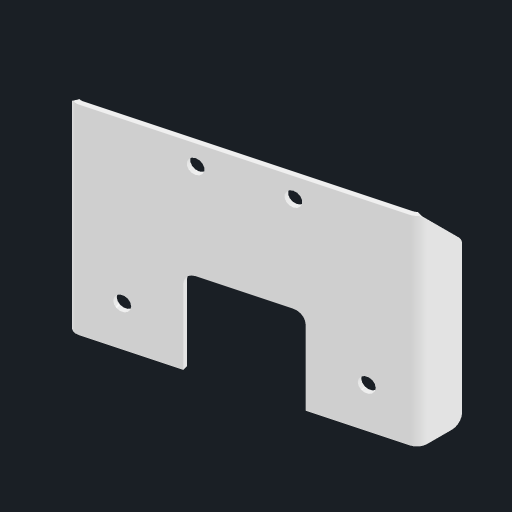
# Autodesk Inventor part: cradle
Saved by Autodesk Inventor 2024.2 (Build 282272000, 272)
## iProperties
Created: 2024-01-06
Part Number: cradle
Material: Generic
Document SubType Name: Sheet Metal
Designer: reima
Density: 1 g/cm^3
Sheet Metal Rule: Default
Appearance: White
Flat Pattern Width: 6.35 cm
Flat Pattern Length: 11.4296 cm
Flat Pattern Area: 72.5782 cm^2
Sheet Metal Width: 2.500 in
Sheet Metal Length: 4.500 in
Sheet Metal Area: 11.250 in^2
Author: reima
Autodesk Inventor part; units mm, degrees
ref_plane "YZ Plane" through (0, 0, 0) normal (1, 0, 0) x (0, 1, 0)
ref_plane "XZ Plane" through (0, 0, 0) normal (0, 1, 0) x (-1, 0, 0)
ref_plane "XY Plane" through (0, 0, 0) normal (0, 0, 1) x (1, 0, 0)
sketch "Sketch1" plane through (0, 0, 0) normal (1, 0, 0) x (0, 1, 0)
  ellipse E0 centre (-29.9633, -76.9903) end of major axis (-32.2747, -76.9903) minor radius 2.3111
  ellipse E1 centre (-29.9633, -102.3866) end of major axis (-32.2747, -102.3866) minor radius 2.3111
  line L0 (-23.6133, -45.2403) -> (-87.1133, -45.2403)
  line L1 (-87.1133, -45.2403) -> (-87.1133, -134.1366)
  line L2 (-87.1133, -134.1366) -> (-23.6133, -134.1366)
  line L3 (-23.6133, -134.1366) -> (-23.6133, -45.2403)
  line L4 (-87.1133, -45.2403) -> (-87.1133, -35.7153)
  line L5 (-87.1133, -45.2403) -> (-77.5883, -45.2403) construction
  line L6 (-23.6133, -45.2403) -> (-35.3834, -33.4702)
  line L7 (-23.6133, -45.2403) -> (-6.9679, -45.2403) construction
  line L8 (-37.6284, -32.5403) -> (-83.9383, -32.5403)
  arc A0 (-83.9383, -32.5403) -> (-87.1133, -35.7153) centre (-83.9383, -35.7153) ccw
  arc A1 (-35.3834, -33.4702) -> (-37.6284, -32.5403) centre (-37.6284, -35.7153) ccw
  line L9 (-87.1133, -89.6885) -> (-23.6133, -89.6885) construction
  line L10 (-87.1133, -134.1366) -> (-87.1133, -143.6616)
  line L11 (-87.1133, -134.1366) -> (-77.5883, -134.1366) construction
  line L12 (-23.6133, -134.1366) -> (-35.3834, -145.9067)
  line L13 (-37.6284, -146.8366) -> (-83.9383, -146.8366)
  arc A2 (-87.1133, -143.6616) -> (-83.9383, -146.8366) centre (-83.9383, -143.6616) ccw
  arc A3 (-37.6284, -146.8366) -> (-35.3834, -145.9067) centre (-37.6284, -143.6616) ccw
  point P0 (0, 0)
  point P1 (-87.1133, -32.5403)
  point P2 (-87.1133, -146.8366)
  dimension "d0" = 6.35
  dimension "d1" = 31.75
  dimension "d2" = 31.75
  dimension "d3" = 63.5
  dimension "d4" = 12.7
  dimension "d5" = 90
  dimension "d6" = 135
  dimension "d7" = 3.175
  measures "d0" distance from line of L3 point (-29.963, -102.387)
  measures "d1" distance from line of point (-29.963, -102.387) L2
  measures "d2" distance from line of point (-29.963, -76.99) L0
  measures "d3" distance between parallel lines of L1 L3
  measures "d4" distance of L0.end point (-87.113, -32.54)
  measures "d5" angle of L5 L4
  measures "d6" angle of L7 L6
  measures "d7" radius of A0
extrude "Plate1" add sketch "Sketch1" along normal blind 1.5875
sketch "Sketch3" plane through (0, 0, 0) normal (-1, 0, 0) x (0, 0, 1)
  ellipse E0 centre (-102.3866, -29.9633) end of major axis (-102.3866, -27.6519) minor radius 2.3111 construction
  ellipse E1 centre (-76.9903, -29.9633) end of major axis (-76.9903, -27.6519) minor radius 2.3111 construction
  arc A0 (-32.5403, -37.6284) -> (-33.4702, -35.3834) centre (-35.7153, -37.6284) ccw construction
  line L0 (-45.2403, -23.6133) -> (-33.4702, -35.3834) construction
  line L1 (-134.1366, -23.6133) -> (-45.2403, -23.6133) construction
  line L2 (-145.9067, -35.3834) -> (-134.1366, -23.6133) construction
  arc A1 (-145.9067, -35.3834) -> (-146.8366, -37.6284) centre (-143.6616, -37.6284) ccw construction
  line L3 (-146.8366, -83.9383) -> (-146.8366, -37.6284) construction
  arc A2 (-146.8366, -83.9383) -> (-143.6616, -87.1133) centre (-143.6616, -83.9383) ccw construction
  line L4 (-35.7153, -87.1133) -> (-143.6616, -87.1133) construction
  arc A3 (-35.7153, -87.1133) -> (-32.5403, -83.9383) centre (-35.7153, -83.9383) ccw construction
  line L5 (-32.5403, -37.6284) -> (-32.5403, -83.9383) construction
  line L6 (-45.2403, -23.6133) -> (-45.2403, -87.1133) construction
  line L7 (-134.1366, -23.6133) -> (-134.1366, -87.1133) construction
  point P0 (0, 0)
  constraints: 4 end point, 2 point on line, 1 perpendicular, 1 vertical
fold "Fold1" angle 75 bend radius 1.5875 thickness 1.5875 k factor 0.44 line from (0, -23.6133, -45.2403) to (0, -87.1133, -45.2403) line at bend centre moving side (0, 0, 1) folds toward (-1, 0, 0)
sketch "Sketch4" plane through (0, 0, 0) normal (-1, 0, 0) x (0, 0, 1)
  line L0 (-46.7365, -87.1133) -> (-46.7365, -23.6133) construction
  line L1 (-134.1366, -23.6133) -> (-46.7365, -23.6133) construction
  line L2 (-145.9067, -35.3834) -> (-134.1366, -23.6133) construction
  arc A0 (-145.9067, -35.3834) -> (-146.8366, -37.6284) centre (-143.6616, -37.6284) ccw construction
  line L3 (-146.8366, -83.9383) -> (-146.8366, -37.6284) construction
  arc A1 (-146.8366, -83.9383) -> (-143.6616, -87.1133) centre (-143.6616, -83.9383) ccw construction
  line L4 (-46.7365, -87.1133) -> (-143.6616, -87.1133) construction
  ellipse E0 centre (-102.3866, -29.9633) end of major axis (-102.3866, -27.6519) minor radius 2.3111 construction
  ellipse E1 centre (-76.9903, -29.9633) end of major axis (-76.9903, -27.6519) minor radius 2.3111 construction
  line L5 (-134.1366, -23.6133) -> (-134.1366, -87.1133)
  point P0 (0, 0)
  constraints: 2 end point, 1 perpendicular, 1 point on line
fold "Fold2" angle 75 bend radius 1.5875 thickness 1.5875 k factor 0.44 line from (0, -23.6133, -134.1366) to (0, -87.1133, -134.1366) line at bend centre moving side (0, 0, 1) folds toward (-1, 0, 0)
sketch "Sketch5" plane through (-1.1766, -87.1133, -134.0994) normal (-0.258819, 0, -0.9659258) x (-0.9659258, 0, 0.258819)
  line L0 (85.904, 0) -> (0, 0) projected
  line L1 (27.0764, 0) -> (58.8264, 0)
  line L2 (58.8264, 0) -> (58.8264, 23.7737)
  line L3 (55.6514, 26.9487) -> (30.2514, 26.9487)
  line L4 (27.0764, 23.7737) -> (27.0764, 0)
  line L5 (0, 63.5) -> (0, 0) projected
  line L6 (58.8264, 26.9487) -> (58.8264, 0)
  line L7 (27.0764, 0) -> (27.0764, 26.9487)
  arc A0 (58.8264, 23.7737) -> (55.6514, 26.9487) centre (55.6514, 23.7737) ccw
  arc A1 (30.2514, 26.9487) -> (27.0764, 23.7737) centre (30.2514, 23.7737) ccw
  point P0 (33.5709, 87.1133)
  dimension "d21" = 31.75
  dimension "d22" = 27.0764
  dimension "d23" = 3.175
  constraints: 12 end point, 5 point on line, 4 point on circle, 4 tangent, 3 parallel, 2 centre point, 1 collinear, 1 equal radius, 1 horizontal, 1 perpendicular
  measures "d21" distance of L7.end L6.start
  measures "d22" distance between parallel lines of L5 L4
  measures "d23" radius of A0
extrude "Cut1" cut sketch "Sketch5" against normal blind 1.5875
sketch "Sketch6" plane through (-84.1535, -87.1133, -111.8658) normal (-0.258819, 0, -0.9659258) x (-0.9659258, 0, 0.258819)
  circle A0 centre (-30.2538, 57.15) radius 2.2225 projected
  circle A1 centre (-55.6501, 57.15) radius 2.2225 projected
  circle A2 centre (-11.2038, 12.7) radius 2.3368
  circle A3 centre (-74.7001, 12.7) radius 2.3368
  point P0 (-52.333, 87.1133)
  dimension "d26" = 4.6736
  dimension "d27" = 19.05
  dimension "d28" = 44.45
  dimension "d29" = 4.6736
  dimension "d30" = 44.45
  dimension "d31" = 19.05
  constraints: 2 centre point
  measures "d26" diameter of A2
  measures "d27" horizontal distance of A2.centre A0.centre
  measures "d28" vertical distance of A0.centre A2.centre
  measures "d29" diameter of A3
  measures "d30" vertical distance of A1.centre A3.centre
  measures "d31" horizontal distance of A1.centre A3.centre
extrude "Cut2" cut sketch "Sketch6" against normal blind 1.5875 contours A2 | A3
equation "\"d8\" = Thickness"
equation "\"d9\" = BendReliefWidth"
equation "\"d10\" = BendReliefDepth"
equation "\"d11\" = MinimumRemnant"
equation "\"d12\" = TransitionRadius"
equation "\"d14\" = BendRadius"
equation "\"d15\" = BendReliefWidth"
equation "\"d16\" = BendReliefDepth"
equation "\"d17\" = MinimumRemnant"
equation "\"d18\" = TransitionRadius"
equation "\"d20\" = BendRadius"
equation "\"d24\" = Thickness"
equation "\"d32\" = Thickness"
equation "\"BendRadius\" = Thickness"
equation "\"BendReliefWidth\" = Thickness"
equation "\"BendReliefDepth\" = 0.5 * Thickness"
equation "\"CornerReliefSize\" = 4 * Thickness"
equation "\"MinimumRemnant\" = 2 * Thickness"
equation "\"TransitionRadius\" = BendRadius"
equation "\"JacobiRadiusSize\" = BendRadius"
equation "\"GapSize\" = Thickness"
equation "\"Thickness\" = 1.5875"
body "Solid1"
